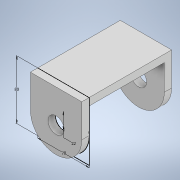
# Autodesk Inventor part: Holder
Saved by Autodesk Inventor 2020 (Build 240168000, 168)
## iProperties
Created: 2020-06-15
Part Number: Holder
Material: Generic
Document SubType Name: Modeling
Designer: jurre
Density: 1 g/cm^3
Appearance: Default
Author: jurre
Autodesk Inventor part; units mm, degrees
ref_plane "YZ Plane" through (0, 0, 0) normal (1, 0, 0) x (0, 1, 0)
ref_plane "XZ Plane" through (0, 0, 0) normal (0, 1, 0) x (-1, 0, 0)
ref_plane "XY Plane" through (0, 0, 0) normal (0, 0, 1) x (1, 0, 0)
sketch "Sketch1" plane through (0, 0, 0) normal (0, 1, 0) x (-1, 0, 0)
  line L0 (35, 51.25) -> (-35, 51.25)
  line L1 (-35, 51.25) -> (-35, -51.25)
  line L2 (-35, -51.25) -> (35, -51.25)
  line L3 (35, -51.25) -> (35, 51.25)
  line L4 (35, 51.25) -> (-35, -51.25) construction
  line L5 (-35, 51.25) -> (35, -51.25) construction
  point P0 (0, 0)
  dimension "d0" = 70
  dimension "d1" = 102.5
  constraints: 12 end point, 2 midpoint, 2 parallel, 1 horizontal, 1 perpendicular
  measures "d0" distance of L0.start L0.end
  measures "d1" distance of L2.end L0.start
extrude "Extrusion1" add sketch "Sketch1" along normal blind 10
sketch "Sketch2" plane through (-35, 0, 51.25) normal (0, 0, 1) x (1, 0, 0)
  line L0 (70, 10) -> (0, 10) projected
  line L1 (0, 10) -> (70, 10)
  line L2 (70, 10) -> (70, -70)
  line L3 (70, -70) -> (0, -70)
  line L4 (0, -70) -> (0, 10)
  circle A0 centre (35, -35) radius 35
  circle A1 centre (35, -35) radius 11
  point P0 (35, 0)
  point P1 (0, -35)
  point P2 (70, -35)
  dimension "d4" = 70
  dimension "d5" = 80
  dimension "d10" = 22
  constraints: 8 end point, 3 tangent, 2 centre point, 2 parallel, 1 coincident, 1 horizontal, 1 perpendicular
  measures "d4" distance of L2.end L3.end
  measures "d5" distance of L3.end L0.end
  measures "d10" diameter of A1
extrude "Extrusion2" add sketch "Sketch2" along normal blind 10 contours L2 A0 L4 L0 | A0
extrude "Extrusion4" add sketch "Sketch2" against normal blind 10 from surface at -102.5 contours L2 A0 L4 L0 | A0
body "Solid1"
